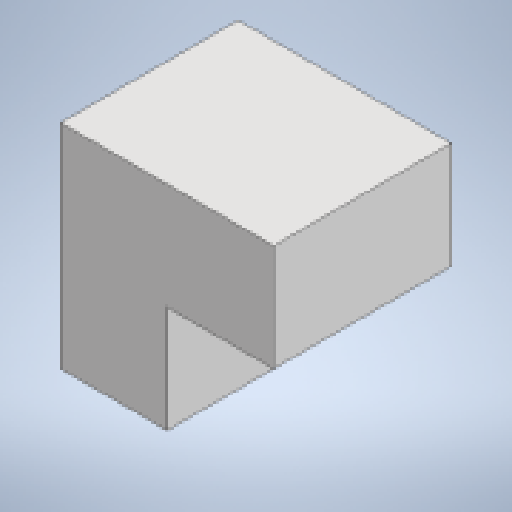
# Autodesk Inventor part: 부품75
Saved by Autodesk Inventor 2024 (Build 280153000, 153)
## iProperties
Created: 2024-09-08
Part Number: 부품75
Material: 일반
Document SubType Name: Modeling
Designer: Eungang
Density: 1 g/cm^3
Appearance: 기본값
Author: Eungang
Autodesk Inventor part; units mm, degrees
ref_plane "YZ Plane" through (0, 0, 0) normal (1, 0, 0) x (0, 1, 0)
ref_plane "XZ Plane" through (0, 0, 0) normal (0, 1, 0) x (-1, 0, 0)
ref_plane "XY Plane" through (0, 0, 0) normal (0, 0, 1) x (1, 0, 0)
sketch "스케치1" plane through (0, 0, 0) normal (0, 0, 1) x (1, 0, 0)
  line L0 (0, 0) -> (63.841, 0) projected
  line L1 (63.841, 0) -> (63.841, 6) projected
  line L2 (0, 6) -> (63.841, 6) projected
  line L3 (0, 0) -> (0, 6) projected
  line L4 (46.0408, 0) -> (46.0408, -150) projected
  line L5 (46.0408, -150) -> (51.8408, -150) projected
  line L6 (51.8408, -150) -> (51.8408, 0) projected
  line L7 (51.8408, 0) -> (46.0408, 0) projected
  line L8 (51.8408, 0) -> (63.841, 0)
  line L9 (63.841, 0) -> (63.841, -6)
  line L10 (63.841, -6) -> (51.8408, -6)
  line L11 (51.8408, -6) -> (51.8408, 0)
  line L12 (57.8409, 0) -> (51.8408, 0)
  line L13 (51.8408, 0) -> (51.8408, -12)
  line L14 (51.8408, -12) -> (57.8409, -12)
  line L15 (57.8409, -12) -> (57.8409, 0)
  point P0 (57.8409, -6)
  constraints: 16 end point, 4 parallel, 2 horizontal, 2 perpendicular, 1 midpoint, 1 point on line
extrude "돌출1" add sketch "스케치1" against normal blind 42 contours L0 L15 L10 L6 | L0 L9 L10 L15 | L10 L15 L14 L6
